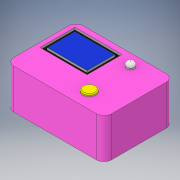
# Autodesk Inventor part: ipt benam
Saved by Autodesk Inventor 2019 (Build 230136000, 136)
## iProperties
Created: 2019-10-21
Part Number: ipt benam
Material: Generic
Document SubType Name: Modeling
Designer: User
Density: 1 g/cm^3
Appearance: Default
Author: User
Autodesk Inventor part; units mm, degrees
ref_plane "YZ Plane" through (0, 0, 0) normal (1, 0, 0) x (0, 1, 0)
ref_plane "XZ Plane" through (0, 0, 0) normal (0, 1, 0) x (-1, 0, 0)
ref_plane "XY Plane" through (0, 0, 0) normal (0, 0, 1) x (1, 0, 0)
sketch "Sketch1" plane through (0, 0, 0) normal (0, 1, 0) x (-1, 0, 0)
  line L0 (3.2051, -3.67) -> (-6.5632, -3.67)
  line L1 (-6.5632, -3.67) -> (-6.5632, -10.643)
  line L2 (-6.5632, -10.643) -> (3.2051, -10.643)
  line L3 (3.2051, -10.643) -> (3.2051, -3.67)
  point P0 (0, 0)
  constraints: 8 end point, 2 parallel, 1 horizontal, 1 perpendicular
extrude "Extrusion1" add sketch "Sketch1" along normal blind 4
sketch "Sketch2" plane through (0, 4, 0) normal (0, 1, 0) x (1, 0, 0)
  line L0 (1.602, 9.7114) -> (1.602, 6.9434)
  line L1 (-2.3871, 6.9434) -> (-2.3871, 9.7114)
  line L2 (-2.7429, 10.0673) -> (-2.7429, 6.5876)
  line L3 (-2.7429, 6.5876) -> (1.9578, 6.5876)
  line L4 (1.9578, 6.5876) -> (1.9578, 10.0673)
  line L5 (-2.3871, 6.9434) -> (1.602, 6.9434)
  line L6 (1.602, 9.7114) -> (-2.3871, 9.7114)
  line L7 (-2.7429, 10.0673) -> (1.9578, 10.0673)
  point P0 (0, 0)
  constraints: 16 end point, 4 parallel, 1 horizontal
extrude "Extrusion2" cut sketch "Sketch2" against normal blind 0.2
sketch "Sketch3" plane through (0, 4, 0) normal (0, 1, 0) x (1, 0, 0)
  circle A0 centre (3.5085, 5.2619) radius 0.6525
  point P0 (0, 0)
  constraints: 1 centre point
extrude "Extrusion3" add sketch "Sketch3" along normal blind 0.2
fillet "Fillet1" radius 0.75 2 edges at (-3.2051, 2, -10.643) (-3.2051, 2, -3.67)
fillet "Fillet2" radius 0.1 1 edges at (2.856, 4.2, -5.2619)
fillet "Fillet3" radius 0.75 1 edges at (6.5632, 2, -10.643)
fillet "Fillet3" radius 0.75 1 edges at (6.5632, 2, -3.67)
sketch "Sketch4" plane through (0, 4, 0) normal (0, 1, 0) x (1, 0, 0)
  circle A0 centre (3.5085, 5.2619) radius 0.5525 projected
  circle A1 centre (3.5085, 5.2619) radius 0.6525 projected
  circle A2 centre (3.4447, 9.4403) radius 0.383
  point P0 (0, 0)
  constraints: 1 centre point
extrude "Extrusion4" add sketch "Sketch4" along normal blind 0.5 contours A2
fillet "Fillet4" radius 0.35 1 edges at (3.0617, 4.5, -9.4403)
body "Solid1"
